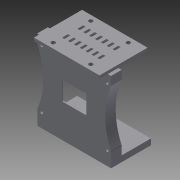
# Autodesk Inventor part: Nikon Base 02
Saved by Autodesk Inventor 2013 (Build 170138000, 138)
## iProperties
Created: 2014-04-13
Part Number: Nikon Base 02
Material: Generic
Document SubType Name: Modeling
Designer: spichelh
Density: 1 g/cm^3
Author: spichelh
Autodesk Inventor part; units mm, degrees
ref_plane "YZ Plane" through (0, 0, 0) normal (1, 0, 0) x (0, 1, 0)
ref_plane "XZ Plane" through (0, 0, 0) normal (0, 1, 0) x (-1, 0, 0)
ref_plane "XY Plane" through (0, 0, 0) normal (0, 0, 1) x (1, 0, 0)
sketch "Sketch1" plane through (0, 0, 0) normal (0, 0, 1) x (1, 0, 0)
  line L0 (0, -8.8929) -> (0, 44.5272) construction
  circle A0 centre (27.94, 24.765) radius 3.5 construction
  circle A1 centre (27.94, 24.765) radius 1.4
  arc A2 (-22.86, 19.685) -> (-22.86, -19.685) centre (-1.3776, 0) ccw construction
  line L1 (-1.3776, 0) -> (-30.5151, 0) construction
  line L2 (-22.86, -19.685) -> (-22.86, -28.575) construction
  circle A3 centre (-27.94, 24.765) radius 3.5 construction
  circle A4 centre (-27.94, 24.765) radius 1.4
  circle A5 centre (-27.94, -24.765) radius 1.4
  circle A6 centre (-27.94, -24.765) radius 3.5 construction
  circle A7 centre (27.94, -24.765) radius 1.4
  circle A8 centre (27.94, -24.765) radius 3.5 construction
  line L3 (-27.94, 24.765) -> (27.94, -24.765) construction
  line L4 (27.94, 24.765) -> (-27.94, -24.765) construction
  line L5 (-22.86, 19.685) -> (-22.86, 28.575) construction
  arc A9 (22.86, -19.685) -> (22.86, 19.685) centre (1.3776, 0) ccw construction
  line L6 (22.86, -19.685) -> (22.86, -28.575) construction
  line L7 (22.86, 19.685) -> (22.86, 28.575) construction
  line L8 (-22.94, 30.575) -> (22.94, 30.575) construction
  line L9 (22.94, 30.575) -> (22.94, -25.765) construction
  line L10 (22.94, -25.765) -> (-22.94, -25.765) construction
  line L11 (-22.94, -25.765) -> (-22.94, 30.575) construction
  line L12 (-50.8, 28.575) -> (50.8, 28.575) construction
  line L13 (50.8, 28.575) -> (50.8, -28.575) construction
  line L14 (50.8, -28.575) -> (-50.8, -28.575) construction
  line L15 (-50.8, -28.575) -> (-50.8, 28.575) construction
  line L16 (-50.8, 28.575) -> (50.8, -28.575) construction
  line L17 (50.8, 28.575) -> (-50.8, -28.575) construction
  arc A10 (-31.1629, -23.4) -> (-31.1629, 23.4) centre (-86.4117, 0) ccw
  line L18 (-31.44, -31.575) -> (-31.44, -24.765)
  line L19 (31.44, -31.575) -> (31.44, -24.765)
  line L20 (-31.44, -31.575) -> (31.44, -31.575)
  arc A11 (-26.1355, -21.7661) -> (-26.1355, 21.7661) centre (-184.648, 0) ccw
  line L21 (-26.1355, -21.7661) -> (-26.1355, -28.575)
  line L22 (26.1355, -28.575) -> (26.1355, -21.7661)
  line L23 (26.1355, -28.575) -> (-26.1355, -28.575)
  line L24 (26.1355, 29.575) -> (26.1355, 21.7661)
  arc A12 (-31.1629, -23.4) -> (-31.44, -24.765) centre (-27.94, -24.765) ccw
  arc A13 (31.44, -24.765) -> (31.1629, -23.4) centre (27.94, -24.765) ccw
  circle A14 centre (27.94, 24.765) radius 1.4
  arc A15 (26.1355, 21.7661) -> (26.1355, -21.7661) centre (184.648, 0) ccw
  line L25 (31.44, 24.765) -> (31.44, 31.575)
  line L26 (-31.44, 31.575) -> (31.44, 31.575)
  line L27 (-31.44, 24.765) -> (-31.44, 31.575)
  line L28 (-26.1355, 21.7661) -> (-26.1355, 29.575)
  line L29 (-26.1355, 29.575) -> (26.1355, 29.575)
  arc A16 (-31.44, 24.765) -> (-31.1629, 23.4) centre (-27.94, 24.765) ccw
  arc A17 (31.1629, 23.4) -> (31.1629, -23.4) centre (86.4117, 0) ccw
  arc A18 (31.1629, 23.4) -> (31.44, 24.765) centre (27.94, 24.765) ccw
  point P0 (0, 0)
  point P1 (0, 0)
  point P2 (0, 0)
  point P3 (0.1677, 29.575)
  dimension "d260" = 1.88
  dimension "d315" = 7
  dimension "d320" = 2.8
  dimension "d325" = 29.1375
  dimension "d327" = 85
  dimension "d328" = 8.89
  dimension "d332" = 55.88
  dimension "d333" = 49.53
  dimension "d334" = 2.8
  dimension "d335" = 7
  dimension "d337" = 5.08
  dimension "d339" = 5
  dimension "d340" = 5
  dimension "d341" = 1
  dimension "d342" = 101.6
  dimension "d343" = 57.15
  dimension "d344" = 2
  dimension "d346" = 60
  dimension "d348" = 6.81
  dimension "d351" = 160
  dimension "d352" = 98.2363
  dimension "d356" = 25.9678
  dimension "d363" = 7
  dimension "d364" = 2.8
  dimension "d366" = 1
  dimension "d367" = 2
  constraints: 60 end point, 27 point on circle, 18 symmetric about line, 17 centre point, 8 parallel, 6 coincident, 6 perpendicular, 5 point on line, 4 midpoint, 4 tangent, 3 horizontal, 3 horizontal alignment, 3 vertical, 2 concentric, 1 line through centre, 1 vertical alignment, 14 other
  measures "d320" diameter of A1
  measures "d325" radius of A2
  measures "d328" distance of L2.start L2.end
  measures "d332" distance of point (27.94, 24.765) A3.centre
  measures "d333" distance of point (-27.94, -24.765) A3.centre
  measures "d334" diameter of A5
  measures "d335" diameter of A6
  measures "d337" distance from line of A5.centre L2
  measures "d339" distance from line of point (27.94, 24.765) L9
  measures "d340" distance from line of A3.centre L11
  measures "d341" distance from line of L10 A7.centre
  measures "d342" distance of L13.end L14.end
  measures "d343" distance of L12.end L13.end
  measures "d344" distance between parallel lines of L12 L8
  measures "d346" radius of A10
  measures "d348" distance of L19.start L19.end
  measures "d351" radius of A11
  measures "d352" distance of A10.centre A11.centre
  measures "d356" distance from line of L24 point (0.168, 29.575)
  measures "d363" diameter of A3
  measures "d364" diameter of A4
  measures "d366" distance between parallel lines of L12 L29
  measures "d367" distance between parallel lines of L26 L29
extrude "Extrusion1" add sketch "Sketch1" along normal blind 9
sketch "Sketch14" plane through (0, 0, 9) normal (0, 0, 1) x (1, 0, 0)
  line L0 (50.88, 56.34) -> (5, 56.34) construction
  line L1 (-22.86, -0.81) -> (78.74, -0.81) construction
  line L2 (-22.86, 56.34) -> (-22.86, -0.81) construction
  line L3 (78.74, -0.81) -> (78.74, 56.34) construction
  circle A0 centre (27.94, 24.765) radius 1.4 projected
  arc A1 (-31.1629, -23.4) -> (-31.44, -24.765) centre (-27.94, -24.765) ccw projected
  line L4 (-31.44, -31.575) -> (31.44, -31.575) projected
  arc A2 (31.44, -24.765) -> (31.1629, -23.4) centre (27.94, -24.765) ccw projected
  line L5 (-27.94, 24.765) -> (27.94, -24.765) construction
  line L6 (-27.94, -24.765) -> (27.94, 24.765) construction
  circle A3 centre (0, 0) radius 23
  line L7 (27.3548, 30.2966) -> (-27.4827, 30.2966)
  line L8 (-27.3618, -29.7074) -> (27.6443, -29.7074)
  line L9 (31.44, 31.575) -> (-31.44, 31.575) projected
  line L10 (-27.4827, 30.2966) -> (-26.4228, 26.165)
  line L11 (-26.4228, 26.165) -> (-26.4228, 23)
  line L12 (-26.4228, 23) -> (-26.4228, 14.1591)
  line L13 (-26.4228, 14.1591) -> (-25.539, 2.7108)
  line L14 (-25.539, 2.7108) -> (-25.9809, -5.703)
  line L15 (-25.9809, -5.703) -> (-26.4228, -19.5882)
  line L16 (-26.4228, -19.5882) -> (-26.341, -23.8125)
  line L17 (-26.341, -23.8125) -> (-26.4338, -26.7299)
  line L18 (-26.4338, -26.7299) -> (-27.3618, -29.7074)
  line L19 (27.6443, -29.7074) -> (26.4117, -25.9501)
  line L20 (26.4117, -25.9501) -> (26.3192, -21.1761)
  line L21 (26.3192, -21.1761) -> (26.1835, -14.1718)
  line L22 (26.1835, -14.1718) -> (25.2275, -1.7896)
  line L23 (25.2275, -1.7896) -> (25.7055, 2.8762)
  line L24 (25.7055, 2.8762) -> (26.4307, 16.6826)
  line L25 (26.4307, 16.6826) -> (26.7625, 23)
  line L26 (26.7625, 23) -> (26.381, 24.487)
  line L27 (26.381, 24.487) -> (26.4419, 26.3982)
  line L28 (26.4419, 26.3982) -> (27.3548, 30.2966)
  dimension "d359" = 46
  constraints: 46 end point, 7 parallel, 3 collinear, 1 centre point, 1 midpoint, 1 perpendicular
  measures "d359" diameter of A3
extrude "Extrusion14" add sketch "Sketch14" against normal blind 2 contours L28 L27 L26 L25 L24 L23 L22 L21 L20 L19 L8 L18 L17 L16 L15 L14 L13 L12 L11 L10 L7
sketch "Sketch17" plane through (0, 0, 7) normal (0, 0, -1) x (-1, 0, 0)
  line L0 (-9.4, 8.05) -> (9.4, 8.05)
  line L1 (10.4, 7.05) -> (10.4, -7.05)
  line L2 (9.4, -8.05) -> (-9.4, -8.05)
  line L3 (-10.4, -7.05) -> (-10.4, 7.05)
  line L4 (10.4, 8.05) -> (-10.4, -8.05) construction
  line L5 (10.4, -8.05) -> (-10.4, 8.05) construction
  circle A0 centre (0, 0) radius 23
  arc A1 (-9.4, 8.05) -> (-10.4, 7.05) centre (-9.4, 7.05) ccw
  arc A2 (-10.4, -7.05) -> (-9.4, -8.05) centre (-9.4, -7.05) ccw
  arc A3 (9.4, -8.05) -> (10.4, -7.05) centre (9.4, -7.05) ccw
  arc A4 (10.4, 7.05) -> (9.4, 8.05) centre (9.4, 7.05) ccw
  dimension "d111" = 20.8
  dimension "d112" = 16.1
  dimension "d115" = 1
  constraints: 12 end point, 8 point on circle, 8 point on line, 8 tangent, 5 centre point, 3 equal radius, 2 coincident, 2 parallel, 1 horizontal, 1 midpoint, 1 perpendicular
  measures "d111" distance of L5.start L4.end
  measures "d112" distance of L4.start L5.start
  measures "d115" radius of A1
extrude "Extrusion17" add sketch "Sketch17" against normal blind 2
sketch "Sketch26" plane through (0, 6, 0) normal (-1, 0, 0) x (0, 0, 1)
  line L0 (0, 43.53) -> (0, 0) projected
  line L1 (-1, 50.34) -> (0, 50.34) construction
  line L2 (-1, -6.81) -> (0, -6.81) construction
  line L3 (4, -6.81) -> (6, -6.81)
  line L4 (6, -6.81) -> (6, 50.34)
  line L5 (6, 50.34) -> (4, 50.34)
  line L6 (4, 50.34) -> (4, -6.81)
  point P0 (0, -6)
  dimension "d140" = 2
  dimension "d141" = 4
  constraints: 8 end point, 2 collinear, 2 parallel, 1 horizontal, 1 perpendicular
  measures "d140" distance of L5.end L4.end
  measures "d141" distance between parallel lines of L0 L6
extrude "Extrusion26" [suppressed]
sketch "Sketch27" plane through (55.88, 6, 0) normal (1, 0, 0) x (0, 0, -1)
  line L0 (1, -6.81) -> (0, -6.81) construction
  line L1 (1, 50.34) -> (0, 50.34) construction
  line L2 (-4, 50.34) -> (-6, 50.34)
  line L3 (-6, 50.34) -> (-6, -6.81)
  line L4 (-6, -6.81) -> (-4, -6.81)
  line L5 (-4, -6.81) -> (-4, 50.34)
  line L6 (0, -13) -> (0, -6) construction
  dimension "d146" = 2
  dimension "d147" = 4
  constraints: 8 end point, 2 collinear, 2 parallel, 1 horizontal, 1 perpendicular
  measures "d146" distance of L4.end L3.end
  measures "d147" distance between parallel lines of L6 L5
extrude "Extrusion27" [suppressed]
sketch "Sketch32" plane through (0, 0, 0) normal (0, 0, -1) x (-1, 0, 0)
  line L0 (-31.44, -36.575) -> (31.44, -36.575)
  line L1 (31.44, -36.575) -> (31.44, -31.575)
  line L2 (31.44, -31.575) -> (-31.44, -31.575)
  line L3 (-31.44, -31.575) -> (-31.44, -36.575)
  line L4 (-31.44, -31.575) -> (31.44, -31.575) projected
  arc A0 (26.1355, 21.7661) -> (26.1355, -21.7661) centre (184.648, 0) ccw projected
  line L5 (26.1355, -21.7661) -> (26.1355, -28.575) projected
  line L6 (26.1355, -28.575) -> (-26.1355, -28.575) projected
  line L7 (-26.1355, -28.575) -> (-26.1355, -21.7661) projected
  arc A1 (-26.1355, -21.7661) -> (-26.1355, 21.7661) centre (-184.648, 0) ccw projected
  line L8 (-26.1355, 21.7661) -> (-26.1355, 29.575) projected
  circle A2 centre (-27.94, -24.765) radius 1.4 projected
  circle A3 centre (27.94, -24.765) radius 1.4 projected
  circle A4 centre (27.94, 24.765) radius 1.4 projected
  circle A5 centre (-27.94, 24.765) radius 1.4 projected
  arc A6 (31.1629, 23.4) -> (31.1629, -23.4) centre (86.4117, 0) ccw projected
  line L9 (31.44, 31.575) -> (-31.44, 31.575) projected
  line L10 (-31.44, 31.575) -> (-31.44, 24.765) projected
  arc A7 (-31.1629, -23.4) -> (-31.44, -24.765) centre (-27.94, -24.765) ccw projected
  line L11 (-31.44, -24.765) -> (-31.44, -31.575) projected
  line L12 (-31.44, -31.575) -> (31.44, -31.575) projected
  line L13 (31.44, -31.575) -> (31.44, -24.765) projected
  arc A8 (31.44, -24.765) -> (31.1629, -23.4) centre (27.94, -24.765) ccw projected
  line L14 (0, -36.575) -> (0, -33.3444) construction
  line L15 (0, -28.575) -> (0, -24.2584) construction
  line L16 (-31.44, -24.765) -> (-31.44, -31.575) projected
  line L17 (26.1355, 29.575) -> (26.1355, 21.7661) projected
  line L18 (-26.1355, 29.575) -> (26.1355, 29.575) projected
  arc A9 (31.1629, 23.4) -> (31.44, 24.765) centre (27.94, 24.765) ccw projected
  line L19 (31.44, 24.765) -> (31.44, 31.575) projected
  arc A10 (-31.44, 24.765) -> (-31.1629, 23.4) centre (-27.94, 24.765) ccw projected
  arc A11 (-31.1629, -23.4) -> (-31.1629, 23.4) centre (-86.4117, 0) ccw projected
  dimension "d180" = 5
  constraints: 12 end point, 4 collinear, 3 parallel, 2 midpoint, 1 horizontal, 1 perpendicular
  measures "d180" distance between parallel lines of L0 L2
extrude "Extrusion32" add sketch "Sketch32" along normal blind 25 and the other way blind 1.5 contours L3 L2 L1 L0
sketch "Sketch35" plane through (-31.44, -36.575, -25) normal (0, -1, 0) x (1, 0, 0)
  line L0 (62.88, 33.8666) -> (0, 33.8666)
  line L1 (0, 33.8666) -> (62.88, 0) construction
  line L2 (62.88, 33.8666) -> (0, 0) construction
  line L3 (31.44, 16.9333) -> (31.44, -14.8721) construction
  circle A0 centre (31.44, 6.9333) radius 3.175
  circle A1 centre (31.44, 18.9333) radius 3.175
  dimension "d194" = 6.35
  dimension "d195" = 10
  dimension "d196" = 6.35
  dimension "d197" = 2
  constraints: 8 end point, 2 centre point, 2 point on line, 2 vertical alignment, 1 horizontal, 1 midpoint, 1 perpendicular
  measures "d194" diameter of A0
  measures "d195" distance of L3.start A0.centre
  measures "d196" diameter of A1
  measures "d197" distance of L3.start A1.centre
extrude "Extrusion34" cut sketch "Sketch35" against normal blind 10
sketch "Sketch37" plane through (52.88, -31.575, 0) normal (0, 1, 0) x (1, 0, 0)
  line L0 (-49.88, -1.5) -> (-49.88, 0) projected
  line L1 (3, -1.5) -> (-52.88, -1.5) projected
  line L2 (0, -1.5) -> (-49.88, -1.5)
  line L3 (-49.88, -1.5) -> (-49.88, 0)
  line L4 (-49.88, 0) -> (0, 0)
  line L5 (0, 0) -> (0, -1.5)
  constraints: 8 end point, 2 parallel, 1 horizontal, 1 perpendicular
extrude "Extrusion36" [suppressed]
sketch "Sketch38" plane through (0, 0, 7) normal (0, 0, -1) x (-1, 0, 0)
  arc A0 (-10.4, -7.05) -> (-9.4, -8.05) centre (-9.4, -7.05) ccw projected
  line L0 (-10.4, -7.05) -> (-10.4, 7.05) projected
  arc A1 (-9.4, 8.05) -> (-10.4, 7.05) centre (-9.4, 7.05) ccw projected
  line L1 (-9.4, 8.05) -> (9.4, 8.05) projected
  arc A2 (10.4, 7.05) -> (9.4, 8.05) centre (9.4, 7.05) ccw projected
  line L2 (10.4, 7.05) -> (10.4, -7.05) projected
  arc A3 (9.4, -8.05) -> (10.4, -7.05) centre (9.4, -7.05) ccw projected
  line L3 (9.4, -8.05) -> (-9.4, -8.05) projected
  line L4 (9.4, 7.05) -> (-9.4, -7.05) construction
  line L5 (9.4, -7.05) -> (-9.4, 7.05) construction
  line L6 (-17.115, 17.115) -> (17.115, 17.115)
  line L7 (17.115, 17.115) -> (17.115, -17.115)
  line L8 (17.115, -17.115) -> (-17.115, -17.115)
  line L9 (-17.115, -17.115) -> (-17.115, 17.115)
  line L10 (17.115, -17.115) -> (-17.115, 17.115) construction
  line L11 (-17.115, -17.115) -> (17.115, 17.115) construction
  point P0 (0, 0)
  point P1 (0, 0)
  dimension "d209" = 34.23
  dimension "d211" = 34.23
  constraints: 16 end point, 3 midpoint, 2 parallel, 1 horizontal, 1 perpendicular
  measures "d209" distance of L8.end L6.start
  measures "d211" distance of L6.start L6.end
extrude "Extrusion37" cut sketch "Sketch38" against normal blind 1
sketch "Sketch39" plane through (0, 0, 8) normal (0, 0, -1) x (-1, 0, 0)
  line L0 (-9.4, -8.05) -> (9.4, -8.05) projected
  arc A0 (-10.4, -7.05) -> (-9.4, -8.05) centre (-9.4, -7.05) ccw projected
  line L1 (-10.4, 7.05) -> (-10.4, -7.05) projected
  arc A1 (-9.4, 8.05) -> (-10.4, 7.05) centre (-9.4, 7.05) ccw projected
  line L2 (9.4, 8.05) -> (-9.4, 8.05) projected
  arc A2 (10.4, 7.05) -> (9.4, 8.05) centre (9.4, 7.05) ccw projected
  line L3 (10.4, -7.05) -> (10.4, 7.05) projected
  arc A3 (9.4, -8.05) -> (10.4, -7.05) centre (9.4, -7.05) ccw projected
  line L4 (-17.115, 17.115) -> (17.115, 17.115) projected
  line L5 (-17.115, -17.115) -> (-17.115, 17.115) projected
  line L6 (17.115, -17.115) -> (-17.115, -17.115) projected
  line L7 (17.115, 17.115) -> (17.115, -17.115) projected
  line L8 (9.4, 7.05) -> (-9.4, -7.05) construction
  line L9 (-9.4, 7.05) -> (9.4, -7.05) construction
  point P0 (0, 0)
  point P1 (0, 0)
  constraints: 4 end point, 1 midpoint
sketch "Sketch40" plane through (0, 0, 9) normal (0, 0, 1) x (1, 0, 0)
  line L0 (-27.2603, 31.575) -> (28.6197, 31.575)
  line L1 (28.6197, 31.575) -> (28.6197, 34.075)
  line L2 (28.6197, 34.075) -> (-27.2603, 34.075)
  line L3 (-27.2603, 34.075) -> (-27.2603, 31.575)
  line L4 (31.44, 31.575) -> (-31.44, 31.575) projected
  line L5 (-30.0799, 31.765) -> (-30.0799, 24.765) projected
  line L6 (0.6797, 34.075) -> (0.6797, 37.7765) construction
  line L7 (0.6797, 31.575) -> (0.6797, 28.075) construction
  point P0 (-31.44, 31.575)
  dimension "d216" = 2.5
  dimension "d217" = 55.88
  constraints: 12 end point, 3 parallel, 2 collinear, 2 horizontal, 1 midpoint, 1 perpendicular, 2 other
  measures "d216" distance of L2.end L0.start
  measures "d217" distance between parallel lines of L3 L1
extrude "Extrusion38" add sketch "Sketch40" along normal blind 7 and the other way blind 34
sketch "Sketch43" plane through (-27.2603, 34.075, 16) normal (0, 1, 0) x (1, 0, 0)
  line L0 (52.88, 24) -> (3, 24)
  line L1 (3, 29) -> (3, 24)
  line L2 (52.88, 29) -> (3, 29)
  line L3 (52.88, 29) -> (52.88, 24)
  line L4 (12, 30) -> (14, 30)
  line L5 (14, 30) -> (14, 25)
  line L6 (14, 25) -> (12, 25)
  line L7 (12, 25) -> (12, 30)
  line L8 (17, 30) -> (19, 30)
  line L9 (19, 30) -> (19, 25)
  line L10 (19, 25) -> (17, 25)
  line L11 (17, 25) -> (17, 30)
  line L12 (22, 30) -> (24, 30)
  line L13 (24, 30) -> (24, 25)
  line L14 (24, 25) -> (22, 25)
  line L15 (22, 25) -> (22, 30)
  line L16 (27, 30) -> (29, 30)
  line L17 (29, 30) -> (29, 25)
  line L18 (29, 25) -> (27, 25)
  line L19 (27, 25) -> (27, 30)
  line L20 (32, 30) -> (34, 30)
  line L21 (34, 30) -> (34, 25)
  line L22 (34, 25) -> (32, 25)
  line L23 (32, 25) -> (32, 30)
  line L24 (37, 30) -> (39, 30)
  line L25 (39, 30) -> (39, 25)
  line L26 (39, 25) -> (37, 25)
  line L27 (37, 25) -> (37, 30)
  line L28 (42, 30) -> (44, 30)
  line L29 (44, 30) -> (44, 25)
  line L30 (44, 25) -> (42, 25)
  line L31 (42, 25) -> (42, 30)
  line L32 (0, 41) -> (0, 0) projected
  line L33 (55.88, 41) -> (55.88, 0) projected
  line L34 (0, 21) -> (55.88, 21) construction
  line L35 (12, 12) -> (14, 12)
  line L36 (14, 12) -> (14, 17)
  line L37 (14, 17) -> (12, 17)
  line L38 (12, 17) -> (12, 12)
  line L39 (19, 12) -> (19, 17)
  line L40 (17, 12) -> (19, 12)
  line L41 (19, 17) -> (17, 17)
  line L42 (24, 12) -> (24, 17)
  line L43 (22, 12) -> (24, 12)
  line L44 (22, 17) -> (22, 12)
  line L45 (24, 17) -> (22, 17)
  line L46 (29, 12) -> (29, 17)
  line L47 (27, 12) -> (29, 12)
  line L48 (27, 17) -> (27, 12)
  line L49 (29, 17) -> (27, 17)
  line L50 (34, 12) -> (34, 17)
  line L51 (32, 12) -> (34, 12)
  line L52 (32, 17) -> (32, 12)
  line L53 (34, 17) -> (32, 17)
  line L54 (39, 12) -> (39, 17)
  line L55 (37, 12) -> (39, 12)
  line L56 (37, 17) -> (37, 12)
  line L57 (39, 17) -> (37, 17)
  line L58 (44, 12) -> (44, 17)
  line L59 (42, 12) -> (44, 12)
  line L60 (42, 17) -> (42, 12)
  line L61 (44, 17) -> (42, 17)
  line L62 (17, 17) -> (17, 12)
  line L63 (55.88, 0) -> (0, 0) projected
  point P0 (0, 27)
  dimension "d233" = 1
  dimension "d234" = 1
  dimension "d235" = 2
  dimension "d236" = 9
  dimension "d239" = 5
  dimension "d295" = 3
  dimension "d296" = 3
  dimension "d297" = 8.88
  dimension "d298" = 5
  dimension "d299" = 21
  constraints: 122 end point, 28 symmetric about line, 2 horizontal, 2 parallel, 2 perpendicular, 2 point on line, 48 other
  measures "d233" distance between parallel lines of L2 L4
  measures "d234" distance between parallel lines of L0 L6
  measures "d235" distance between parallel lines of L7 L5
  measures "d236" distance between parallel lines of L7 L1
  measures "d239" distance of L4.end L9.start
  measures "d295" distance between parallel lines of L32 L1
  measures "d296" distance between parallel lines of L33 L3
  measures "d297" distance between parallel lines of L3 L29
  measures "d298" distance between parallel lines of L8 L10
  measures "d299" distance between parallel lines of L63 L34
extrude "Extrusion41" cut sketch "Sketch43" against normal blind 5 contours L29 L30 L31 L2 | L2 L31 L28 L29 | L7 L4 L5 L2 | L2 L5 L6 L7 | L25 L26 L27 L2 | L2 L27 L24 L25 | L11 L8 L9 L2 | L2 L9 L10 L11 | L21 L22 L23 L2 | L2 L23 L20 L21 | L15 L12 L13 L2 | L2 L13 L14 L15 | L17 L18 L19 L2 | L2 L19 L16 L17 | L38 L37 L36 L35 | L40 L62 L41 L39 | L43 L44 L45 L42 | L47 L48 L49 L46 | L51 L52 L53 L50 | L55 L56 L57 L54 | L59 L60 L61 L58
sketch "Sketch44" plane through (-26.1355, -28.575, 0) normal (0, 1, 0) x (1, 0, 0)
  line L0 (49.88, -7.5) -> (0, -7.5)
  line L1 (0, -7.5) -> (0, 0)
  line L2 (0, 0) -> (49.88, 0)
  line L3 (49.88, -7.5) -> (49.88, 0)
  line L4 (2, -1) -> (4, -1)
  line L5 (4, -1) -> (4, -6.5)
  line L6 (4, -6.5) -> (2, -6.5)
  line L7 (2, -6.5) -> (2, -1)
  line L8 (7.5, -1) -> (9.5, -1)
  line L9 (9.5, -1) -> (9.5, -6.5)
  line L10 (9.5, -6.5) -> (7.5, -6.5)
  line L11 (7.5, -6.5) -> (7.5, -1)
  line L12 (13, -1) -> (15, -1)
  line L13 (15, -1) -> (15, -6.5)
  line L14 (15, -6.5) -> (13, -6.5)
  line L15 (13, -6.5) -> (13, -1)
  line L16 (18.5, -1) -> (20.5, -1)
  line L17 (20.5, -1) -> (20.5, -6.5)
  line L18 (20.5, -6.5) -> (18.5, -6.5)
  line L19 (18.5, -6.5) -> (18.5, -1)
  line L20 (24, -1) -> (26, -1)
  line L21 (26, -1) -> (26, -6.5)
  line L22 (26, -6.5) -> (24, -6.5)
  line L23 (24, -6.5) -> (24, -1)
  line L24 (29.5, -1) -> (31.5, -1)
  line L25 (31.5, -1) -> (31.5, -6.5)
  line L26 (31.5, -6.5) -> (29.5, -6.5)
  line L27 (29.5, -6.5) -> (29.5, -1)
  line L28 (35, -1) -> (37, -1)
  line L29 (37, -1) -> (37, -6.5)
  line L30 (37, -6.5) -> (35, -6.5)
  line L31 (35, -6.5) -> (35, -1)
  line L32 (40.5, -1) -> (42.5, -1)
  line L33 (42.5, -1) -> (42.5, -6.5)
  line L34 (42.5, -6.5) -> (40.5, -6.5)
  line L35 (40.5, -6.5) -> (40.5, -1)
  line L36 (46, -1) -> (48, -1)
  line L37 (48, -1) -> (48, -6.5)
  line L38 (48, -6.5) -> (46, -6.5)
  line L39 (46, -6.5) -> (46, -1)
  point P0 (0, -9)
  dimension "d247" = 1
  dimension "d248" = 1
  dimension "d249" = 2
  dimension "d250" = 2
  dimension "d253" = 5.5
  dimension "d260" = 1.88
  constraints: 80 end point, 2 horizontal, 2 parallel, 1 perpendicular, 64 other
  measures "d247" distance between parallel lines of L2 L4
  measures "d248" distance between parallel lines of L0 L6
  measures "d249" distance between parallel lines of L7 L5
  measures "d250" distance between parallel lines of L1 L7
  measures "d253" distance of L4.end L9.start
  measures "d260" distance between parallel lines of L37 L3
extrude "Extrusion42" cut sketch "Sketch44" against normal blind 5 contours L4 L5 L6 L7 | L8 L9 L10 L11 | L12 L13 L14 L15 | L16 L17 L18 L19 | L20 L21 L22 L23 | L24 L25 L26 L27 | L28 L29 L30 L31 | L32 L33 L34 L35 | L36 L37 L38 L39
sketch "Sketch46" plane through (-27.2603, 34.075, 16) normal (0, 1, 0) x (1, 0, 0)
  circle A0 centre (11.94, 36.5) radius 1.7
  circle A1 centre (43.94, 36.5) radius 1.7
  line L0 (43.94, 36.5) -> (11.94, 36.5) construction
  circle A2 centre (43.94, 4.5) radius 1.7
  line L1 (0, 41) -> (0, 0) projected
  line L2 (55.88, 0) -> (0, 0) projected
  line L3 (55.88, 41) -> (55.88, 0) projected
  line L4 (0, 41) -> (55.88, 41) projected
  line L5 (55.88, 20.5) -> (0, 20.5) construction
  line L6 (27.94, 41) -> (27.94, 0) construction
  line L7 (43.94, 4.5) -> (43.94, 36.5) construction
  circle A3 centre (11.94, 4.5) radius 1.7
  point P0 (27.94, 36.5)
  point P1 (43.94, 20.5)
  dimension "d275" = 3.4
  dimension "d277" = 3.4
  dimension "d278" = 32
  dimension "d279" = 32
  dimension "d294" = 3.4
  constraints: 8 end point, 6 midpoint, 4 centre point, 2 point on line, 1 horizontal, 1 symmetric about line, 1 other
  measures "d275" diameter of A0
  measures "d277" diameter of A1
  measures "d278" distance of L0.start L0.end
  measures "d279" distance of L7.start L0.start
  measures "d294" diameter of A2
extrude "Extrusion44" cut sketch "Sketch46" against normal blind 5 contours A0 | A1 | A2 | A3
sketch "Sketch49" plane through (0, 0, 0) normal (0, 0, -1) x (-1, 0, 0)
  line L0 (0, 55.53) -> (0, 58.53) projected
  line L1 (-55.88, 58.53) -> (0, 58.53)
  line L2 (0, 58.53) -> (0, 56.53)
  line L3 (0, 56.53) -> (-55.88, 56.53)
  line L4 (-55.88, 56.53) -> (-55.88, 58.53)
  constraints: 8 end point, 2 parallel, 1 horizontal, 1 perpendicular, 1 point on line
extrude "Extrusion46" [suppressed]
sketch "Sketch51" plane through (0, 0, 7) normal (0, 0, -1) x (-1, 0, 0)
  line L0 (17.115, -17.115) -> (-17.115, -17.115) projected
  line L1 (-3, -2.5) -> (-52.88, -2.5) projected
  line L2 (-37.44, -2.5) -> (-35.44, -2.5)
  line L3 (-35.44, -2.5) -> (-35.44, 0.5)
  line L4 (-35.44, 0.5) -> (-37.44, 0.5)
  line L5 (-37.44, 0.5) -> (-37.44, -2.5)
  line L6 (-27.94, -2.5) -> (-27.94, -17.115) construction
  line L7 (-31.94, -2.5) -> (-29.94, -2.5)
  line L8 (-29.94, -2.5) -> (-29.94, 0.5)
  line L9 (-29.94, 0.5) -> (-31.94, 0.5)
  line L10 (-31.94, 0.5) -> (-31.94, -2.5)
  line L11 (-26.44, -2.5) -> (-24.44, -2.5)
  line L12 (-24.44, -2.5) -> (-24.44, 0.5)
  line L13 (-24.44, 0.5) -> (-26.44, 0.5)
  line L14 (-26.44, 0.5) -> (-26.44, -2.5)
  line L15 (-20.94, -2.5) -> (-18.94, -2.5)
  line L16 (-18.94, -2.5) -> (-18.94, 0.5)
  line L17 (-18.94, 0.5) -> (-20.94, 0.5)
  line L18 (-20.94, 0.5) -> (-20.94, -2.5)
  point P0 (0, 0)
  dimension "d300" = 0
  dimension "d301" = 2
  dimension "d302" = 3
  dimension "d303" = 15
  dimension "d308" = 5.5
  constraints: 34 end point, 2 horizontal, 2 parallel, 1 midpoint, 1 perpendicular, 1 point on line, 24 other
  measures "d300" distance between parallel lines of L2 L1
  measures "d301" distance of L2.start L2.end
  measures "d302" distance between parallel lines of L4 L2
  measures "d303" diameter of L3 L6
  measures "d308" distance of L3.end L9.start
extrude "Extrusion48" [suppressed]
sketch "Sketch52" plane through (0, 0, 1.5) normal (0, 0, 1) x (1, 0, 0)
  line L0 (-31.44, -36.575) -> (31.44, -36.575) projected
  line L1 (31.44, -36.575) -> (31.44, -31.575) projected
  line L2 (-31.44, -31.575) -> (31.44, -31.575) projected
  line L3 (-31.44, -31.575) -> (-31.44, -36.575) projected
  line L4 (-31.44, -36.575) -> (31.44, -36.575) projected
  line L5 (31.44, -36.575) -> (31.44, -31.575) projected
  line L6 (-31.44, -31.575) -> (-24.1355, -31.575) projected
  line L7 (-31.44, -31.575) -> (-31.44, -36.575) projected
  line L8 (14.3645, -33.575) -> (14.3645, -31.575) projected
  line L9 (10.8645, -31.575) -> (14.3645, -31.575) projected
  line L10 (10.8645, -31.575) -> (10.8645, -33.575) projected
  line L11 (10.8645, -33.575) -> (8.8645, -33.575) projected
  line L12 (8.8645, -33.575) -> (8.8645, -31.575) projected
  line L13 (5.3645, -31.575) -> (8.8645, -31.575) projected
  line L14 (5.3645, -31.575) -> (5.3645, -33.575) projected
  line L15 (5.3645, -33.575) -> (3.3645, -33.575) projected
  line L16 (3.3645, -33.575) -> (3.3645, -31.575) projected
  line L17 (-0.1355, -31.575) -> (3.3645, -31.575) projected
  line L18 (-0.1355, -31.575) -> (-0.1355, -33.575) projected
  line L19 (-0.1355, -33.575) -> (-2.1355, -33.575) projected
  line L20 (-2.1355, -33.575) -> (-2.1355, -31.575) projected
  line L21 (-5.6355, -31.575) -> (-2.1355, -31.575) projected
  line L22 (-5.6355, -31.575) -> (-5.6355, -33.575) projected
  line L23 (-5.6355, -33.575) -> (-7.6355, -33.575) projected
  line L24 (-7.6355, -33.575) -> (-7.6355, -31.575) projected
  line L25 (-11.1355, -31.575) -> (-7.6355, -31.575) projected
  line L26 (-11.1355, -31.575) -> (-11.1355, -33.575) projected
  line L27 (-11.1355, -33.575) -> (-13.1355, -33.575) projected
  line L28 (-13.1355, -33.575) -> (-13.1355, -31.575) projected
  line L29 (-16.6355, -31.575) -> (-13.1355, -31.575) projected
  line L30 (-16.6355, -31.575) -> (-16.6355, -33.575) projected
  line L31 (-16.6355, -33.575) -> (-18.6355, -33.575) projected
  line L32 (-18.6355, -33.575) -> (-18.6355, -31.575) projected
  line L33 (-22.1355, -31.575) -> (-18.6355, -31.575) projected
  line L34 (-22.1355, -31.575) -> (-22.1355, -33.575) projected
  line L35 (-22.1355, -33.575) -> (-24.1355, -33.575) projected
  line L36 (-24.1355, -33.575) -> (-24.1355, -31.575) projected
  line L37 (21.8645, -31.575) -> (31.44, -31.575) projected
  line L38 (21.8645, -31.575) -> (21.8645, -33.575) projected
  line L39 (21.8645, -33.575) -> (19.8645, -33.575) projected
  line L40 (19.8645, -33.575) -> (19.8645, -31.575) projected
  line L41 (16.3645, -31.575) -> (19.8645, -31.575) projected
  line L42 (16.3645, -31.575) -> (16.3645, -33.575) projected
  line L43 (16.3645, -33.575) -> (14.3645, -33.575) projected
  point P0 (0, 0)
extrude "Extrusion49" add sketch "Sketch52" along normal blind 7.5
body "Solid1"
